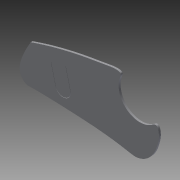
# Autodesk Inventor part: pickGuard02
Saved by Autodesk Inventor 2013 (Build 170138000, 138)
## iProperties
Created: 2014-04-22
Part Number: pickGuard02
Material: Generic
Document SubType Name: Modeling
Designer: Nano
Density: 1 g/cm^3
Author: Nano
Autodesk Inventor part; units mm, degrees
ref_plane "YZ Plane" through (0, 0, 0) normal (1, 0, 0) x (0, 1, 0)
ref_plane "XZ Plane" through (0, 0, 0) normal (0, 1, 0) x (-1, 0, 0)
ref_plane "XY Plane" through (0, 0, 0) normal (0, 0, 1) x (1, 0, 0)
sketch "Sketch1" plane through (0, 0, 0) normal (0, 0, 1) x (1, 0, 0)
  arc A0 (99.0804, 37.7819) -> (99.0369, 37.6475) centre (132.2899, 26.9707) ccw
  spline S0 degree 2 poles (58.7626, 42.8458) (4.0618, 34.0895) (-47.5552, 16.3255) knots 0 0 0 1 1 1
  spline S1 degree 4 poles (-47.5552, 16.3255) (-55.7268, 2.159) (-55.4543, 1.5771) (-66.9192, -18.8164) (-67.6496, -39.0914) (-57.5491, -47.1396) (-52.1718, -47.8438) knots 0 0 0 0 0 0.392924 0.642924 1 1 1 1 1
  line L0 (-27.7337, 50.6881) -> (-67.3766, -18.0371) construction
  arc A1 (-31.3128, 43.5784) -> (-63.0141, -11.3794) centre (916.5156, -539.7802) ccw construction
  line L1 (-68.5865, -45.6943) -> (-35.7572, -49.9933) construction
  arc A2 (-59.5605, -42.8684) -> (-43.7512, -44.9387) centre (-50.8755, -37.9448) ccw construction
  spline S2 degree 4 poles (58.7626, 42.8458) (92.5705, 48.8541) (69.1224, 44.4272) (107.1274, 52.6766) (100.7874, 42.9522) (99.0358, 37.6479) knots 0 0 0 0 0 0.552252 1 1 1 1 1
  line L2 (46.0358, 40.584) -> (71.4894, 45.1076) construction
  arc A3 (68.945, 44.65) -> (48.5821, 41.0311) centre (1808.5325, -9802.8794) ccw construction
  line L3 (100.5127, 42.1206) -> (97.5589, 33.1752) construction
  arc A4 (100.4221, 41.1299) -> (98.076, 34.025) centre (128.7331, 27.8415) ccw construction
  spline S3 degree 4 poles (-52.1718, -47.8438) (-29.2578, -46.9791) (12.1287, -49.4902) (72.3754, -50.4308) (122.3026, -61.1787) (126.0487, -61.2077) (141.7651, -57.3615) (156.328, -42.5827) (160.8678, -26.8681) (164.7227, -14.9795) (163.1481, -1.3758) (159.0756, 3.6288) (153.5971, -0.703) (153.3806, -0.867) knots 0 0 0 0 0 0.281182 0.407801 0.508909 0.558199 0.615243 0.695069 0.768301 0.853871 0.920208 1 1 1 1 1
  line L4 (-73.5152, -48.6492) -> (-30.8285, -47.0384) construction
  arc A5 (-35.1153, -47.7859) -> (-69.1843, -49.0715) centre (-42.8001, -296.1961) ccw construction
  line L5 (110.453, -62.1891) -> (142.2724, -59.2716) construction
  arc A6 (115.5464, -58.4524) -> (136.5843, -56.5234) centre (124.6496, -42.0465) ccw construction
  line L6 (121.2218, -72.5663) -> (169.0186, -32.8418) construction
  arc A7 (124.9955, -61.6613) -> (157.6074, -34.5572) centre (119.1641, -21.4734) ccw construction
  line L7 (156.4177, 1.434) -> (150.3434, -3.1681) construction
  arc A8 (152.0082, -0.9418) -> (153.824, 0.4339) centre (152.639, 0.1118) ccw construction
  line L8 (99.0369, 37.6475) -> (153.3777, -0.865) construction
  arc A9 (99.0369, 37.6475) -> (153.3806, -0.867) centre (132.2899, 26.9707) ccw
  arc A10 (99.6942, 39.5117) -> (99.0804, 37.7819) centre (132.2899, 26.9707) ccw
  arc A11 (153.3806, -0.867) -> (99.6942, 39.5117) centre (132.2899, 26.9707) ccw
  point P0 (4.6365, 31.7886)
  point P1 (-57.8731, -2.8569)
  point P2 (-64.386, -19.8711)
  point P3 (-63.6674, -38.8819)
  point P4 (88.0143, 47.7336)
  point P5 (99.9346, 46.3882)
  point P6 (28.3047, -49.9527)
  point P7 (109.7614, -58.564)
  point P8 (126.3627, -60.7303)
  point P9 (145.1202, -52.704)
  point P10 (160.7409, -27.4895)
  point P11 (163.7264, -11.9433)
  point P12 (161.4453, -0.8489)
  point P13 (157.2479, 1.1365)
  dimension "d0" = 69.85
  constraints: 18 end point, 16 midpoint, 16 point on circle, 12 centre point, 2 tangent, 1 point on line, 38 other
  measures "d0" diameter of A0
extrude "Extrusion1" add sketch "Sketch1" along normal blind 3.175 contours A0 A9 S3 S1 S0 S2 A10
sketch "Sketch2" plane through (0, 0, 3.175) normal (0, 0, 1) x (1, 0, 0)
  circle A0 centre (15.7533, 91.0014) radius 114.3 construction
  line L0 (5.6398, -22.8503) -> (-15.867, 63.409) construction
  line L1 (5.6398, -22.8503) -> (94.5398, -22.8503) construction
  line L2 (-6.6829, -25.9227) -> (5.6398, -22.8503) construction
  line L3 (-6.6829, -25.9227) -> (-5.1635, -25.8417)
  line L4 (17.9626, -19.7779) -> (10.36, 10.7144)
  arc A1 (-6.6829, -25.9227) -> (17.9626, -19.7779) centre (5.6398, -22.8503) ccw
  line L5 (-12.8707, -27.4655) -> (40.4255, -14.1773) construction
  arc A2 (-6.19, -25.7998) -> (17.4697, -19.9008) centre (5.6398, -22.8503) ccw
  line L6 (9.8671, 10.5915) -> (10.36, 10.7144)
  line L7 (-13.7926, 4.6925) -> (-14.2855, 4.5696)
  line L8 (-6.6829, -25.9227) -> (-14.2855, 4.5696)
  line L9 (10.36, 10.7144) -> (10.36, 10.7144)
  line L10 (-6.19, -25.7998) -> (-13.7926, 4.6925)
  line L11 (17.4697, -19.9008) -> (9.8671, 10.5915)
  point P0 (0, 0)
  point P1 (-6.6829, -25.9227)
  dimension "d7" = 35
  dimension "d3" = 228.6
  dimension "d14" = 88.9
  dimension "d15" = 104
  dimension "d17" = 25.4
  dimension "d18" = 31.75
  dimension "d19" = 0.508
  constraints: 24 end point, 4 point on circle, 3 centre point, 3 parallel, 3 point on line, 3 symmetric about line, 1 coincident, 1 equal length, 1 horizontal, 1 other
  measures "d3" diameter of A0
  measures "d14" distance of L0.start L0.end
  measures "d15" angle of L1 L0
  measures "d17" diameter of A1
  measures "d18" distance of L3.end L7.end
  measures "d19" radial gap between concentric circles of A1 A2
extrude "Extrusion2" cut sketch "Sketch2" against normal up to next
body "Solid1"
